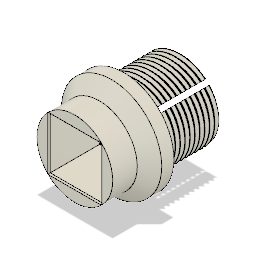
55part (Autodesk Fusion 360 design; units mm, degrees)
Autodesk Fusion 360 part; units mm, degrees
sketch "Sketch1" plane through (0, 0, 0) normal (0, 1, 0) x (1, 0, 0)
  line L0 (16, 43) -> (16, 20)
  line L1 (16, 20) -> (20.5, 20)
  line L2 (20.5, 20) -> (20.5, 15)
  line L3 (20.5, 15) -> (15.5, 10)
  line L4 (15.5, 10) -> (15.5, 0)
  line L5 (15.5, 0) -> (0, 0)
  line L6 (16, 43) -> (0, 43)
  line L7 (0, 43) -> (0, 0)
  dimension "d2" = 16
  dimension "d3" = 15.5
  dimension "d4" = 10
  dimension "d5" = 5
  dimension "d17" = 23
  dimension "d100" = 5
  dimension "d101" = 10
  constraint vertical L0
  constraint perpendicular L0 L1
  constraint perpendicular L1 L2
  constraint perpendicular L2 L5
  constraint perpendicular L0 L6
  constraint perpendicular L5 L7
  constraint coincident L5.end L7.end
  constraint vertical L4
  measures "d2" distance of L0.start L6.end
  measures "d3" distance of L4.end L5.end
  measures "d4" distance of L3.end L4.end
  measures "d5" distance of L1.end L2.end
  measures "d17" distance of L0.start L0.end
  measures "d100" distance of L2 L4
  measures "d101" distance of L1 L3.end
revolve "Revolve2" add sketch "Sketch1" angle 360 about axis through (0, 0, -205.75) along (0, 0, 1)
sketch "Sketch23" plane through (0, 0, 0) normal (0, 0, 1) x (1, 0, 0)
  circle A0 centre (0, 0) radius 15.5
  line L0 (10.5, 10.5) -> (-10.5, 10.5)
  line L1 (-10.5, 10.5) -> (-10.5, -10.5)
  line L2 (-10.5, -10.5) -> (10.5, -10.5)
  line L3 (10.5, -10.5) -> (10.5, 10.5)
  line L4 (10.5, 10.5) -> (-10.5, -10.5) construction
  line L5 (-10.5, 10.5) -> (10.5, -10.5) construction
  dimension "d51" = 21
  dimension "d54" = 21
  constraint perpendicular L0 L1
  constraint parallel L0 L2
  constraint parallel L1 L3
  constraint horizontal L0
  constraint coincident L4 A0.centre
  constraint coincident L5 A0.centre
  constraint coincident A0.centre origin
  measures "d51" distance of L0.end L1.end
  measures "d54" distance of L1.end L2.end
extrude "Extrude5" cut sketch "Sketch23" against normal up to surface (43 mm away) contours L0 L1 L2 L3
thread "Thread2" "ISO Metric profile 32.0 M32x2 6g" major diameter 31.822 minor diameter 29.5289 pitch 2 angle 60 modelled right hand crest width 0.25 on face at (15.9801, -0.7975, -35.3333) crest through (15.911, 0, -43.125)
sketch "Sketch11" plane through (0, 0, -43) normal (0, 0, -1) x (-1, 0, 0)
  spline S0 degree 3 poles (14.2033, 4.0317) (13.7448, 5.9115) (12.9211, 7.6828) (10.6286, 10.8358) (9.1734, 12.1809) (5.8079, 14.2569) (3.9246, 14.9588) (-0.0321, 15.6107) (-2.0691, 15.5442) (-5.3755, 14.7836) (-6.6675, 14.3004) (-9.1044, 13.0055) (-10.2372, 12.1964) (-11.2508, 11.2508) knots 0 0 0 0 0.580476 0.580476 1.169153 1.169153 1.766027 1.766027 2.371098 2.371098 2.782632 2.782632 3.197913 3.197913 3.197913 3.197913
  arc A0 (-11.2508, 11.2508) -> (-15.911, 0) centre (0, 0) ccw
  spline S1 degree 3 poles (-15.911, 0) (-15.8398, -2.0558) (-15.3703, -4.0781) (-13.6892, -7.8018) (-12.5035, -9.4715) (-9.5752, -12.2398) (-7.8682, -13.3192) (-4.1602, -14.7484) (-2.199, -15.0941) (1.0838, -15.0233) (2.385, -14.8239) (4.8897, -14.0933) (6.0831, -13.5684) (7.1924, -12.8941) knots 0 0 0 0 0.617113 0.617113 1.226021 1.226021 1.826722 1.826722 2.419212 2.419212 2.812944 2.812944 3.202923 3.202923 3.202923 3.202923
  line L0 (15.2028, -13.7886) -> (-13.7886, 15.2028)
  line L1 (-13.7886, 15.2028) -> (-15.2028, 13.7886)
  line L2 (-15.2028, 13.7886) -> (13.7886, -15.2028)
  line L3 (13.7886, -15.2028) -> (15.2028, -13.7886)
  line L4 (-13.9187, -15.0838) -> (15.3207, 13.6574)
  line L5 (-15.3207, -13.6574) -> (-13.9187, -15.0838)
  line L6 (13.9187, 15.0838) -> (-15.3207, -13.6574)
  line L7 (15.3207, 13.6574) -> (13.9187, 15.0838)
  arc A1 (7.1924, -12.8941) -> (10.3797, -10.5) centre (0, 0) ccw
  circle A2 centre (0, 0) radius 20.5
  line L8 (10.3797, -10.5) -> (-10.5, -10.5)
  line L9 (-10.5, -10.5) -> (-10.5, 10.5)
  line L10 (-10.5, 10.5) -> (10.5, 10.5)
  line L11 (10.5, 10.5) -> (10.5, -10.3797)
  arc A3 (10.5, -10.3797) -> (14.2033, 4.0317) centre (0, 0) ccw
  constraint perpendicular L0 L1
  constraint parallel L0 L2
  constraint parallel L1 L3
  constraint coincident A0.centre A1.centre
  constraint perpendicular L4 L7
  constraint parallel L4 L6
  constraint parallel L5 L7
  constraint tangent L5 A2
  constraint tangent L3 A2
  constraint tangent L7 A2
  constraint tangent L1 A2
extrude "Extrude4" cut sketch "Sketch11" against normal blind 20 contours S0 L4 L6 L10 L11 | S0 L4 L6 A2 | L0 L11 A3 | L0 L2 L4 A1 A2 L8 L11 A3 | L0 L4 L6 L10 L11 | L4 L7 A2 | L0 L3 A2 | S0 A0 L0 L2 L9 L10 | S0 A0 L0 L2 A2 | L6 L7 A2 | L2 L3 A2 | L0 L2 L6 L9 L10 | L0 L1 A2 | L2 L4 L6 L8 L9 | L1 L2 A2 | L2 A1 L8 | S1 L4 L6 L8 L9 | S1 L4 L6 A2 | L4 L5 A2 | L5 L6 A2
chamfer "Chamfer2" distance 0.5 angle 45 8 edges at (-0.0848, 10.5, -43) (-10.5, -0.0835, -43) (0.0848, -10.5, -43) (10.5, 0.0835, -43) (10.5, 0, 0) (0, 10.5, 0) (0, -10.5, 0) (-10.5, 0, 0)
equation "d54 = d51"
